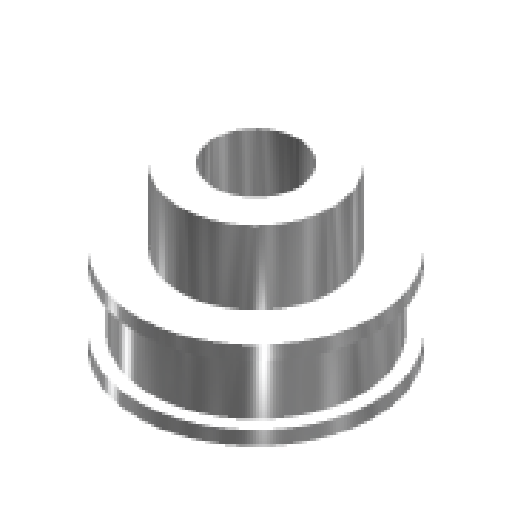
# Autodesk Inventor part: Z Axis Belt Pulley
Saved by Autodesk Inventor 2023.2 (Build 272271000, 271)
## iProperties
Created: 2023-02-17
Part Number: Z Axis Belt Pulley
Material: Aluminum 6061
Document SubType Name: Modeling
Designer: remop
Density: 2.7 g/cm^3
Appearance: Aluminum - Flat
Author: remop
Autodesk Inventor part; units mm, degrees
ref_plane "YZ Plane" through (0, 0, 0) normal (1, 0, 0) x (0, 1, 0)
ref_plane "XZ Plane" through (0, 0, 0) normal (0, 1, 0) x (-1, 0, 0)
ref_plane "XY Plane" through (0, 0, 0) normal (0, 0, 1) x (1, 0, 0)
sketch "Sketch1" plane through (0, 0, 0) normal (1, 0, 0) x (0, 1, 0)
  line L0 (0, 0) -> (19, 0)
  line L1 (19, 0) -> (19, -9)
  line L2 (19, -9) -> (10.3, -9)
  line L3 (10.3, -9) -> (10.3, -14)
  line L4 (10.3, -14) -> (8.65, -14)
  line L5 (8.65, -14) -> (8.65, -12.5)
  line L6 (8.65, -12.5) -> (1.65, -12.5)
  line L7 (1.65, -12.5) -> (1.65, -14)
  line L8 (1.65, -14) -> (0, -14)
  line L9 (0, -14) -> (0, 0)
  line L10 (0, -5) -> (19, -5)
  point P0 (14.65, -9)
  point P1 (9.5, -5)
  dimension "d0" = 19
  dimension "d1" = 18
  dimension "d2" = 28
  dimension "d3" = 7
  dimension "d4" = 8.7
  dimension "d5" = 10
  dimension "d6" = 25
  constraints: 22 end point, 9 perpendicular, 4 point on line, 2 midpoint, 1 collinear, 1 horizontal
  measures "d0" distance of L0.start L0.end
  measures "d1" diameter of point (14.65, -9) L0
  measures "d2" diameter of L8 L0
  measures "d3" distance of L5.end L6.end
  measures "d4" distance of L1.end L2.end
  measures "d5" diameter of point (9.5, -5) L0
  measures "d6" diameter of L6 L0
revolve "Revolution1" add sketch "Sketch1" angle 360 about axis through (0, 0, 0) along (0, 1, 0) contours L10 L1 L2 L3 L4 L5 L6 L7 L8 L9
body "Solid1"
